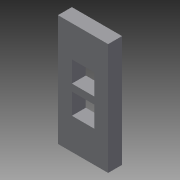
# Autodesk Inventor part: ShortSupportRod
Saved by Autodesk Inventor 2013 (Build 170138000, 138)
## iProperties
Created: 2013-01-18
Part Number: ShortSupportRod
Material: Generic
Document SubType Name: Modeling
Designer: motoennies
Density: 1 g/cm^3
Author: motoennies
Autodesk Inventor part; units mm, degrees
ref_plane "YZ Plane" through (0, 0, 0) normal (1, 0, 0) x (0, 1, 0)
ref_plane "XZ Plane" through (0, 0, 0) normal (0, 1, 0) x (-1, 0, 0)
ref_plane "XY Plane" through (0, 0, 0) normal (0, 0, 1) x (1, 0, 0)
sketch "Sketch1" plane through (0, 0, 0) normal (0, 0, 1) x (1, 0, 0)
  line L0 (0, 0) -> (0, 50.8)
  line L1 (0, 0) -> (22.86, 0)
  line L2 (22.86, 0) -> (22.86, 50.8)
  line L3 (22.86, 50.8) -> (0, 50.8)
  line L4 (6.35, 36.5125) -> (16.51, 36.5125)
  line L5 (6.35, 36.5125) -> (6.35, 26.9875)
  line L6 (6.35, 26.9875) -> (16.51, 26.9875)
  line L7 (16.51, 26.9875) -> (16.51, 36.5125)
  line L8 (0, 25.4) -> (22.86, 25.4) construction
  line L9 (6.35, 14.2875) -> (16.51, 14.2875)
  line L10 (6.35, 14.2875) -> (6.35, 23.8125)
  line L11 (6.35, 23.8125) -> (16.51, 23.8125)
  line L12 (16.51, 23.8125) -> (16.51, 14.2875)
  dimension "d0" = 50.8
  dimension "d1" = 22.86
  dimension "d2" = 10.16
  dimension "d3" = 14.2875
  dimension "d5" = 9.525
  dimension "d6" = 6.35
  constraints: 26 end point, 4 perpendicular, 4 symmetric about line, 3 parallel, 2 midpoint, 1 vertical
  measures "d0" distance of L0.start L0.end
  measures "d1" distance of L0.start L1.end
  measures "d2" distance of L4.start L4.end
  measures "d3" distance between parallel lines of L3 L4
  measures "d5" distance of L4.start L5.end
  measures "d6" distance between parallel lines of L2 L7
extrude "Extrusion1" add sketch "Sketch1" along normal blind 6.35
body "Solid1"
